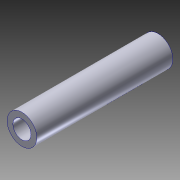
# Autodesk Inventor part: PulleyShaft
Saved by Autodesk Inventor 2013 (Build 170138000, 138)
## iProperties
Created: 2013-11-09
Part Number: PulleyShaft
Material: Generic
Document SubType Name: Modeling
Designer: JustinIndra
Density: 1 g/cm^3
Author: JustinIndra
Autodesk Inventor part; units mm, degrees
ref_plane "YZ Plane" through (0, 0, 0) normal (1, 0, 0) x (0, 1, 0)
ref_plane "XZ Plane" through (0, 0, 0) normal (0, 1, 0) x (-1, 0, 0)
sketch "Sketch1" plane through (0, 0, 0) normal (0, 1, 0) x (-1, 0, 0)
  circle A0 centre (0, 0) radius 2.45
  circle A1 centre (0, 0) radius 1.5
  dimension "d0" = 4.9
  dimension "d1" = 3
  constraints: 2 centre point, 2 coincident
  measures "d0" diameter of A0
  measures "d1" diameter of A1
extrude "Extrusion1" add sketch "Sketch1" along normal mid plane 22.5
ref_plane "Work Plane1" through (0, 0, -2.45) normal (0, 0, 1) x (1, 0, 0)
sketch "Sketch2" plane through (0, 0, -2.45) normal (0, 0, 1) x (1, 0, 0)
  line L0 (2.5, 7.25) -> (-2.5, 7.25)
  line L1 (-2.5, 7.25) -> (-2.5, 1.25)
  line L2 (-2.5, 1.25) -> (2.5, 1.25)
  line L3 (2.5, 1.25) -> (2.5, 7.25)
  line L4 (2.45, 11.25) -> (-2.45, 11.25) projected
  point P0 (0, 0)
  point P1 (0, 7.25)
  dimension "d4" = 6
  dimension "d6" = 4
  dimension "d7" = 5
  constraints: 8 end point, 2 parallel, 1 horizontal, 1 midpoint, 1 perpendicular, 1 vertical alignment
  measures "d4" distance of L0.end L1.end
  measures "d6" distance between parallel lines of L4 L0
  measures "d7" distance of L1.end L2.end
extrude "Extrusion2" cut sketch "Sketch2" along normal blind 0.5
body "Solid1"
